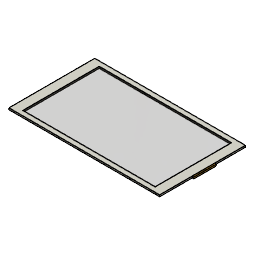
xkcd Comic Reader Case (Autodesk Fusion 360 archive; units mm, degrees)
design "Screen"
Autodesk Fusion 360 part; units mm, degrees
sketch "Sketch1" plane through (0, 0, 0) normal (0, 0, 1) x (1, 0, 0)
  line L0 (-55, 50, 1) -> (38, 50, 1)
  line L1 (38, 50, 1) -> (38, -3, 1)
  line L2 (38, -3, 1) -> (-55, -3, 1)
  line L3 (-55, -3, 1) -> (-55, 50, 1)
  line L4 (32.27, -0.02, 1) -> (-49.27, -0.02, 1)
  line L5 (-49.27, -0.02, 1) -> (-49.27, 47.02, 1)
  line L6 (-49.27, 47.02, 1) -> (32.27, 47.02, 1)
  line L7 (32.27, 47.02, 1) -> (32.27, -0.02, 1)
  point P0 (-8.5, 23.5)
  dimension "d1" = 93
  dimension "d2" = 53
  dimension "d3" = 81.54
  dimension "d4" = 47.04
extrude "Extrude1" add sketch "Sketch1" against normal blind 1 contours L4 L5 L6 L7 in plane through (0, 0, 1) normal (0, 0, 1) makes body 1
extrude "Extrude3" add sketch "Sketch1" against normal blind 1 separate body contours L0 L1 L2 L3 in plane through (0, 0, 1) normal (0, 0, 1) makes body 2
sketch "Sketch3" plane through (38, 0, 0) normal (1, 0, 0) x (0, 1, 0)
  line L0 (50, 1) -> (-3, 1)
  line L1 (-3, 1) -> (-3, 0)
  line L2 (-3, 0) -> (50, 0)
  line L3 (50, 0) -> (50, 1)
  line L4 (50, 1) -> (30.86, 1)
  line L5 (30.86, 1) -> (17.06, 1)
  line L6 (17.06, 1) -> (17.06, 0)
  line L7 (17.06, 0) -> (30.86, 0)
  line L8 (30.86, 0) -> (30.86, 1)
  dimension "d15" = 19.14
  dimension "d16" = 13.8
  dimension "d17" = 1
  constraint coincident L0.start L3.end
  constraint perpendicular L3 L4
  constraint horizontal L5
  constraint vertical L6
  constraint horizontal L7
  constraint vertical L8
  measures "d15" distance of L0.start L4.end
  measures "d16" distance of L4.end L5.end
  measures "d17" distance of L4.end L7.end
extrude "Extrude4" add sketch "Sketch3" along normal blind 1 separate body contours L0 L2 L5 L6 L7 L8 makes body 3
named bodies: "Screen", "Screen Body", "Cable"
